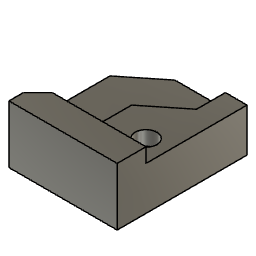
Design 1 (Autodesk Fusion 360 design; units mm, degrees)
Autodesk Fusion 360 part; units mm, degrees
sketch "Sketch1" plane through (0, 0, 0) normal (0, 0, 1) x (1, 0, 0) in component "block"
  line L0 (0, 0) -> (75, 0)
  line L1 (75, 0) -> (75, 75)
  line L2 (75, 75) -> (75, 90)
  line L3 (0, 0) -> (0, 70)
  line L4 (0, 70) -> (25, 90)
  line L5 (25, 90) -> (75, 90)
  constraint coincident L0.start L3.start
  constraint horizontal L0
  constraint perpendicular L0 L1
  constraint perpendicular L0 L2
  constraint perpendicular L0 L3
  constraint perpendicular L2 L5
extrude "Extrude1" add sketch "Sketch1" along normal blind 20 in component "block"
sketch "Sketch2" plane through (0, 0, 20) normal (0, 0, 1) x (-1, 0, 0) in component "block"
  line L0 (0, 0) -> (-75, 0)
  line L1 (-75, 0) -> (-75, -90)
  line L2 (-75, -90) -> (-25, -90)
  line L3 (-25, -90) -> (0, -70)
  line L4 (0, -70) -> (0, 0)
  line L5 (-75, -20) -> (-35, -20)
  line L6 (-35, -20) -> (-35, -50)
  line L7 (-35, -50) -> (-60, -70)
  line L8 (-60, -70) -> (-60, -90)
  constraint coincident L1 L5.start
  constraint perpendicular L1 L5
  constraint perpendicular L5 L6
  constraint coincident L2 L8.end
  constraint perpendicular L2 L8
extrude "Extrude2" add sketch "Sketch2" along normal blind 10 contours L1 L2 L5 L6 L7 L8 in component "block"
sketch "Sketch3" plane through (0, 0, 20) normal (0, 0, 1) x (-1, 0, 0) in component "block"
  line L0 (-60, -70) -> (-60, -90)
  line L1 (-60, -90) -> (-25, -90)
  line L2 (-25, -90) -> (0, -70)
  line L3 (0, -70) -> (0, 0)
  line L4 (0, 0) -> (-75, 0)
  line L5 (-75, 0) -> (-75, -20)
  line L6 (-75, -20) -> (-35, -20)
  line L7 (-35, -20) -> (-35, -50)
  line L8 (-35, -50) -> (-60, -70)
  line L9 (-35, -20) -> (-10, -20)
  line L10 (-10, -20) -> (0, -10)
  constraint coincident L6.end L7.start
  constraint perpendicular L3 L9
  constraint coincident L3 L10.end
extrude "Extrude3" add sketch "Sketch3" along normal blind 20 contours L3 L4 L5 L6 L9 L10 in component "block"
sketch "Sketch4" plane through (0, 0, 30) normal (0, 0, 1) x (-1, 0, 0) in component "block"
  line L0 (-75, -20) -> (-75, -90)
  line L1 (-75, -90) -> (-60, -90)
  line L2 (-60, -90) -> (-60, -70)
  line L3 (-60, -70) -> (-35, -50)
  line L4 (-35, -50) -> (-35, -20)
  line L5 (-35, -20) -> (-75, -20)
  circle A0 centre (-60, -35) radius 7.5
  dimension "d7" = 15
  measures "d7" diameter of A0
extrude "Extrude4" cut sketch "Sketch4" against normal blind 10 contours A0 in component "block"
sketch "Sketch5" plane through (0, 20, 0) normal (0, 1, 0) x (-1, 0, 0) in component "block"
  line L0 (-75, 30) -> (-35, 30)
  line L1 (-35, 30) -> (-35, 20)
  line L2 (-35, 20) -> (-10, 20)
  line L3 (-10, 20) -> (-10, 40)
  line L4 (-10, 40) -> (-75, 40)
  line L5 (-75, 40) -> (-75, 30)
  circle A0 centre (-25, 30) radius 7.5
  dimension "d11" = 15
  measures "d11" diameter of A0
extrude "Extrude5" cut sketch "Sketch5" against normal blind 10 contours A0 in component "block"
component "block" placed x (1, 0, 0) y (0, 1, 0) z (0, 0, 1) at (0, 0, 0)
